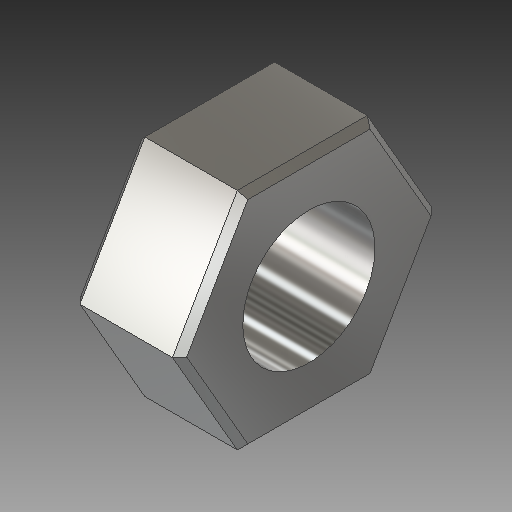
# Autodesk Inventor part: 04-01-Гайка М10
Saved by Autodesk Inventor 2018 (Build 220112000, 112)
## iProperties
Part Number: 04-01-Гайка М10
Material: Типовые
Document SubType Name: Modeling
Designer: sbnnl
Density: 1 g/cm^3
Appearance: Хром - полированный
Author: sbnnl
Autodesk Inventor part; units mm, degrees
ref_plane "YZ Plane" through (0, 0, 0) normal (1, 0, 0) x (0, 1, 0)
ref_plane "XZ Plane" through (0, 0, 0) normal (0, 1, 0) x (-1, 0, 0)
ref_plane "XY Plane" through (0, 0, 0) normal (0, 0, 1) x (1, 0, 0)
sketch "Эскиз1" plane through (0, 0, 0) normal (1, 0, 0) x (0, 1, 0)
  line L0 (0, -9.815) -> (-8.5, -4.9075)
  line L1 (-8.5, -4.9075) -> (-8.5, 4.9075)
  line L2 (-8.5, 4.9075) -> (0, 9.815)
  line L3 (0, 9.815) -> (8.5, 4.9075)
  line L4 (8.5, 4.9075) -> (8.5, -4.9075)
  line L5 (8.5, -4.9075) -> (0, -9.815)
  circle A0 centre (0, 0) radius 5
  dimension "d0" = 17
  dimension "d1" = 10
  constraints: 12 end point, 2 coincident, 1 centre point, 1 vertical, 13 other
  measures "d0" distance between parallel lines of L1 L4
  measures "d1" diameter of A0
extrude "Выдавливание1" add sketch "Эскиз1" along normal blind 8
chamfer "Фаска1" distance 0.5 angle 45 12 edges at (8, 4.25, 7.3612) (8, 8.5, 0) (8, 4.25, -7.3612) (8, -4.25, -7.3612) (8, -8.5, 0) (8, -4.25, 7.3612) (0, 4.25, 7.3612) (0, -4.25, 7.3612) (0, 8.5, 0) (0, 4.25, -7.3612) (0, -4.25, -7.3612) (0, -8.5, 0)
